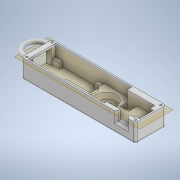
# Autodesk Inventor part: RespiraCheck-Enclosure-Top
Saved by Autodesk Inventor 2022 (Build 260153000, 153)
## iProperties
Created: 2022-04-28
Part Number: RespiraCheck-Enclosure-Top
Material: Generic
Document SubType Name: Modeling
Designer: incep
Density: 1 g/cm^3
Appearance: Default
Author: incep
Autodesk Inventor part; units mm, degrees
ref_plane "YZ Plane" through (0, 0, 0) normal (1, 0, 0) x (0, 1, 0)
ref_plane "XZ Plane" through (0, 0, 0) normal (0, 1, 0) x (-1, 0, 0)
ref_plane "XY Plane" through (0, 0, 0) normal (0, 0, 1) x (1, 0, 0)
sketch "Sketch1" plane through (0, 0, 0) normal (0, 1, 0) x (-1, 0, 0)
  line L0 (56, 15) -> (-56, 15)
  line L1 (-56, 15) -> (-56, -15)
  line L2 (-56, -15) -> (56, -15)
  line L3 (56, -15) -> (56, 15)
  point P0 (0, 0)
  point P1 (-56, 0)
  point P2 (0, -15)
  dimension "d0" = 30
  dimension "d1" = 112
  constraints: 8 end point, 2 midpoint, 2 parallel, 1 horizontal, 1 horizontal alignment, 1 perpendicular, 1 vertical alignment
  measures "d0" distance of L2.end L0.start
  measures "d1" distance of L1.end L2.end
extrude "Extrusion1" add sketch "Sketch1" along normal blind 19
sketch "Sketch2" plane through (0, 19, 0) normal (0, 1, 0) x (1, 0, 0)
  circle A0 centre (-53.5, 12.5) radius 2.5 construction
  line L0 (56, 15) -> (-56, 15) construction
  line L1 (-56, 15) -> (-56, -15) construction
  circle A1 centre (-53.5, -12.5) radius 2.5 construction
  circle A2 centre (53.5, 12.5) radius 2.5 construction
  circle A3 centre (53.5, -12.5) radius 2.5 construction
  line L2 (-56, -15) -> (56, -15) construction
  line L3 (56, -15) -> (56, 15) construction
  line L4 (-51, 13.6) -> (-3, 13.6)
  line L5 (-3, -13.6) -> (-51, -13.6)
  line L6 (-51, -13.6) -> (-51, 13.6)
  line L7 (-3, 8) -> (0, 8)
  line L8 (0, 8) -> (0, -8)
  line L9 (0, -8) -> (-3, -8)
  line L10 (-3, -8) -> (-3, 8) construction
  line L11 (-3, 8) -> (0, 5)
  line L12 (-3, -8) -> (0, -5)
  line L13 (-3, 13.6) -> (-3, 8)
  line L14 (-3, -8) -> (-3, -13.6)
  circle A4 centre (-53.5, 12.5) radius 1
  circle A5 centre (-53.5, -12.5) radius 1
  circle A6 centre (53.5, 12.5) radius 1
  circle A7 centre (53.5, -12.5) radius 1
  point P0 (0, 0)
  point P1 (-2, 0)
  point P2 (0, 0)
  point P3 (-51, 0)
  dimension "d4" = 5
  dimension "d5" = 5
  dimension "d6" = 5
  dimension "d7" = 5
  dimension "d8" = 27.2
  dimension "d10" = 3
  dimension "d11" = 16
  dimension "d14" = 48
  dimension "d15" = 45
  dimension "d16" = 45
  dimension "d64" = 2
  dimension "d65" = 2
  dimension "d66" = 2
  dimension "d67" = 2
  constraints: 22 end point, 9 tangent, 8 centre point, 5 coincident, 5 parallel, 3 perpendicular, 2 collinear, 2 horizontal, 2 midpoint, 2 point on line, 1 horizontal alignment
  measures "d4" diameter of A0
  measures "d5" diameter of A1
  measures "d6" diameter of A2
  measures "d7" diameter of A3
  measures "d8" distance of L5.end L4.start
  measures "d10" distance of L7.start L7.end
  measures "d11" distance of L7.end L8.end
  measures "d14" distance between parallel lines of L6 L13
  measures "d15" angle of L7 L11
  measures "d16" angle of L9 L12
  measures "d64" diameter of A4
  measures "d65" diameter of A5
  measures "d66" diameter of A6
  measures "d67" diameter of A7
extrude "Extrusion2" cut sketch "Sketch2" against normal blind 11.5 contours L4 L13 L11 L8 L12 L14 L5 L6 | A4 | A5 | A6 | A7
sketch "Sketch3" plane through (0, 7.5, 0) normal (0, 1, 0) x (1, 0, 0)
  line L0 (-3, 10) -> (-3, -10)
  line L1 (-51, -10) -> (-51, 10)
  line L2 (-51, -13.6) -> (-51, 13.6) projected
  line L3 (-3, 13.6) -> (-3, 8) projected
  line L4 (-10, -10) -> (-10, -13.6)
  line L5 (-10, -13.6) -> (-44, -13.6)
  line L6 (-44, -13.6) -> (-44, -10)
  line L7 (-3, -8) -> (-3, -13.6) projected
  line L8 (-3, -10) -> (-10, -10)
  line L9 (-44, -10) -> (-51, -10)
  line L10 (-51, 10) -> (-44, 10)
  line L11 (-10, 10) -> (-3, 10)
  line L12 (-51, 13.6) -> (-3, 13.6) projected
  line L13 (-9, 10) -> (-9, 13.6)
  line L14 (-9, 13.6) -> (-44, 13.6)
  line L15 (-44, 13.6) -> (-44, 10)
  point P0 (0, 0)
  point P1 (-3, 0)
  point P2 (-44, 13.6)
  dimension "d20" = 7
  dimension "d21" = 7
  constraints: 24 end point, 7 parallel, 3 point on line, 2 collinear, 2 horizontal, 2 perpendicular, 1 horizontal alignment, 1 midpoint
  measures "d20" distance between parallel lines of L4 L7
  measures "d21" distance between parallel lines of L2 L6
extrude "Extrusion3" cut sketch "Sketch3" against normal blind 5.5 contours L0 L8 L4 L5 L6 L9 L1 L10 L15 L12 L13 L11
sketch "Sketch4" plane through (0, 2, 0) normal (0, 1, 0) x (1, 0, 0)
  line L0 (-32, 5.1) -> (-8, 5.1)
  line L1 (-8, 5.1) -> (-8, -8.9)
  line L2 (-8, -8.9) -> (-32, -8.9)
  line L3 (-32, -8.9) -> (-32, 5.1)
  line L4 (-3, 8) -> (-3, -8) projected
  line L5 (-51, 13.6) -> (-3, 13.6) projected
  line L6 (-3, -13.6) -> (-51, -13.6) projected
  point P0 (0, 0)
  dimension "d24" = 5
  dimension "d25" = 8.5
  dimension "d26" = 4.7
  dimension "d27" = 24
  constraints: 8 end point, 2 parallel, 1 horizontal, 1 perpendicular
  measures "d24" distance between parallel lines of L4 L1
  measures "d25" distance between parallel lines of L0 L5
  measures "d26" distance between parallel lines of L6 L2
  measures "d27" distance between parallel lines of L3 L1
extrude "Extrusion4" cut sketch "Sketch4" against normal blind 2
sketch "Sketch5" plane through (0, 19, 0) normal (0, 1, 0) x (1, 0, 0)
  line L0 (-51, 13.6) -> (-3, 13.6) projected
  line L1 (-3, 13.6) -> (24, 13.6)
  line L2 (24, 13.6) -> (24, -13.6)
  line L3 (24, -13.6) -> (-3, -13.6)
  line L4 (-3, -13.6) -> (-3, 13.6)
  circle A0 centre (53.5, 12.5) radius 2.5 construction
  circle A1 centre (53.5, -12.5) radius 2.5 construction
  line L5 (-3, -13.6) -> (-51, -13.6) projected
  line L6 (0, 5) -> (0, -5) projected
  point P0 (0, 0)
  dimension "d43" = 24
  constraints: 8 end point, 2 parallel, 1 collinear, 1 horizontal, 1 perpendicular
  measures "d43" distance between parallel lines of L2 L6
extrude "Extrusion5" cut sketch "Sketch5" against normal blind 10.5
sketch "Sketch6" plane through (0, 8.5, 0) normal (0, 1, 0) x (1, 0, 0)
  circle A0 centre (12, 0) radius 10.1
  line L0 (0, -5) -> (0, 5) projected
  point P0 (0, 0)
  dimension "d32" = 20.2
  dimension "d33" = 12
  constraints: 1 centre point, 1 horizontal alignment
  measures "d32" diameter of A0
  measures "d33" distance from line of L0 A0.centre
extrude "Extrusion6" cut sketch "Sketch6" against normal blind 6.5
sketch "Sketch7" plane through (12, 2, 0) normal (0, 1, 0) x (1, 0, 0)
  circle A0 centre (0, 0) radius 10.1 projected
  circle A1 centre (0, 0) radius 6.5
  point P0 (-12, 0)
  dimension "d36" = 13
  constraints: 1 centre point, 1 coincident
  measures "d36" diameter of A1
extrude "Extrusion7" cut sketch "Sketch7" against normal blind 2 contours A1
sketch "Sketch8" plane through (0, 19, 0) normal (0, 1, 0) x (1, 0, 0)
  line L0 (24, 9.15) -> (51.1, 9.15)
  line L1 (51.1, 9.15) -> (51.1, -11.15)
  line L2 (51.1, -11.15) -> (24, -11.15)
  line L3 (24, -11.15) -> (24, 9.15)
  circle A0 centre (12, 0) radius 10.1 projected
  line L4 (24, -1) -> (51.1, -1) construction
  line L5 (24, 13.6) -> (24, -13.6) projected
  line L6 (51.1, 4.35) -> (54.6, 4.35)
  line L7 (54.6, 4.35) -> (54.6, -9.65)
  line L8 (54.6, -9.65) -> (51.1, -9.65)
  line L9 (51.1, -9.65) -> (51.1, 4.35)
  point P0 (0, 0)
  dimension "d39" = 20.3
  dimension "d42" = 1
  dimension "d46" = 27.1
  dimension "d47" = 14
  dimension "d48" = 3.5
  dimension "d49" = 1.5
  constraints: 18 end point, 4 parallel, 2 collinear, 2 horizontal, 2 midpoint, 2 perpendicular
  measures "d39" distance of L2.end L0.start
  measures "d42" vertical distance of L4.start A0.centre
  measures "d46" distance between parallel lines of L1 L3
  measures "d47" distance of L6.end L7.end
  measures "d48" distance of L6.start L6.end
  measures "d49" distance from line of L1.end L8
extrude "Extrusion8" cut sketch "Sketch8" against normal blind 9 contours L0 L1 L2 L3 | L6 L7 L8 L1
sketch "Sketch9" plane through (0, 10, 0) normal (0, 1, 0) x (1, 0, 0)
  line L0 (24, 9.15) -> (34, 9.15)
  line L1 (34, 9.15) -> (34, 0.15)
  line L2 (34, 0.15) -> (24, 0.15)
  line L3 (24, 0.15) -> (24, 9.15)
  line L4 (24, 9.15) -> (51.1, 9.15) projected
  line L5 (24, -11.15) -> (24, 9.15) projected
  point P0 (0, 0)
  dimension "d50" = 10
  dimension "d51" = 9
  constraints: 8 end point, 2 collinear, 2 parallel, 1 horizontal, 1 perpendicular
  measures "d50" distance of L1.end L2.end
  measures "d51" distance of L0.end L1.end
extrude "Extrusion9" cut sketch "Sketch9" against normal blind 10.5
sketch "Sketch10" plane through (51.1, 19, 11.15) normal (0, 0, -1) x (-1, 0, 0)
  line L0 (4, 0) -> (14, 0)
  line L1 (14, 0) -> (14, -9)
  line L2 (14, -9) -> (4, -9)
  line L3 (4, -9) -> (4, 0)
  line L4 (0, 0) -> (0, -9) projected
  line L5 (0, 0) -> (27.1, 0) projected
  line L6 (0, -9) -> (27.1, -9) projected
  point P0 (51.1, -19)
  dimension "d54" = 4
  dimension "d55" = 10
  constraints: 8 end point, 2 collinear, 2 parallel, 1 horizontal, 1 perpendicular
  measures "d54" distance between parallel lines of L4 L3
  measures "d55" distance between parallel lines of L1 L3
extrude "Extrusion10" cut sketch "Sketch10" against normal through all contours L0 L1 L2 L3
sketch "Sketch11" plane through (-56, 0, -15) normal (-1, 0, 0) x (0, 0, 1)
  line L0 (6, 17) -> (24, 17)
  line L1 (24, 17) -> (24, 2)
  line L2 (24, 2) -> (6, 2)
  line L3 (6, 2) -> (6, 17)
  line L4 (30, 0) -> (30, 19) projected
  line L5 (0, 0) -> (0, 19) projected
  line L6 (0, 0) -> (30, 0) projected
  line L7 (0, 19) -> (30, 19) projected
  point P0 (15, 0)
  dimension "d58" = 6
  dimension "d59" = 6
  dimension "d60" = 2
  dimension "d61" = 2
  constraints: 8 end point, 2 parallel, 1 horizontal, 1 perpendicular
  measures "d58" distance between parallel lines of L4 L1
  measures "d59" distance between parallel lines of L5 L3
  measures "d60" distance between parallel lines of L6 L2
  measures "d61" distance between parallel lines of L7 L0
extrude "Extrusion11" cut sketch "Sketch11" against normal up to surface (5 mm away) contours L0 L1 L2 L3
sketch "Sketch12" plane through (0, 0, 0) normal (0, -1, 0) x (1, 0, 0)
  line L0 (-45.861, -11.1947) -> (-45.861, 30.7358) construction
  line L1 (-45.861, 30.7358) -> (-41.9267, 30.7358) construction
  line L2 (-41.9267, 30.7358) -> (-41.9267, -11.1947) construction
  line L3 (-41.9267, -11.1947) -> (-45.861, -11.1947) construction
  line L4 (-43.2644, -9.2745) -> (-44.1875, -9.9511)
  spline S0 degree 2 poles (-44.1875, -9.9511) (-44.274, -9.6153) (-44.6708, -9.2974) (-44.9632, -9.2974) knots 0 0 0 1 2 2 2
  spline S1 degree 2 poles (-44.9632, -9.2974) (-45.154, -9.2974) (-45.4693, -9.4322) (-45.5787, -9.5619) knots 0 0 0 1 2 2 2
  spline S2 degree 2 poles (-45.5787, -9.5619) (-45.6804, -9.6789) (-45.7644, -9.9943) (-45.7644, -10.2435) knots 0 0 0 1 2 2 2
  line L5 (-45.7644, -10.2435) -> (-45.7644, -10.9633)
  line L6 (-45.7644, -10.9633) -> (-43.2644, -10.9633)
  line L7 (-43.2644, -10.9633) -> (-43.2644, -10.5004)
  line L8 (-43.2644, -10.5004) -> (-44.2232, -10.5004)
  line L9 (-44.2232, -10.5004) -> (-43.2644, -9.8468)
  line L10 (-43.2644, -9.8468) -> (-43.2644, -9.2745)
  spline S3 degree 2 poles (-44.9505, -9.7654) (-44.7521, -9.7629) (-44.569, -10.007) (-44.5716, -10.274) knots 0 0 0 1 2 2 2
  line L11 (-44.5716, -10.274) -> (-44.5716, -10.5004)
  line L12 (-44.5716, -10.5004) -> (-45.3218, -10.5004)
  line L13 (-45.3218, -10.5004) -> (-45.3218, -10.2944)
  spline S4 degree 2 poles (-45.3218, -10.2944) (-45.3218, -10.0782) (-45.2277, -9.8468) (-45.0624, -9.7629) (-44.9505, -9.7654) knots 0 0 0 1 2 3 3 3
  spline S5 degree 2 poles (-44.1748, -7.1764) (-44.4673, -7.1789) (-44.92, -7.4282) (-45.1794, -7.8631) (-45.182, -8.1454) knots 0 0 0 1 2 3 3 3
  spline S6 degree 2 poles (-45.182, -8.1454) (-45.1794, -8.4226) (-44.9175, -8.8676) (-44.4749, -9.1296) (-44.1952, -9.1321) knots 0 0 0 1 2 3 3 3
  spline S7 degree 2 poles (-44.1952, -9.1321) (-43.918, -9.1296) (-43.4805, -8.8625) (-43.2237, -8.4073) (-43.2211, -8.1174) knots 0 0 0 1 2 3 3 3
  spline S8 degree 2 poles (-43.2211, -8.1174) (-43.2211, -7.9266) (-43.3585, -7.5655) (-43.6255, -7.2908) (-43.8188, -7.2247) knots 0 0 0 1 2 3 3 3
  line L14 (-43.8188, -7.2247) -> (-43.8188, -7.7155)
  spline S9 degree 2 poles (-43.8188, -7.7155) (-43.7196, -7.7995) (-43.6331, -7.9902) (-43.6331, -8.1276) knots 0 0 0 1 2 2 2
  spline S10 degree 2 poles (-43.6331, -8.1276) (-43.6357, -8.331) (-43.8315, -8.6031) (-44.0019, -8.6464) knots 0 0 0 1 2 2 2
  line L15 (-44.0019, -8.6464) -> (-44.0019, -7.1942)
  spline S11 degree 2 poles (-44.0019, -7.1942) (-44.0477, -7.184) (-44.1265, -7.1764) (-44.1748, -7.1764) knots 0 0 0 1 2 2 2
  line L16 (-44.3986, -7.6214) -> (-44.3986, -8.6591)
  spline S12 degree 2 poles (-44.3986, -8.6591) (-44.5792, -8.6057) (-44.77, -8.3386) (-44.77, -8.1377) knots 0 0 0 1 2 2 2
  spline S13 degree 2 poles (-44.77, -8.1377) (-44.77, -7.9292) (-44.5792, -7.6647) (-44.3986, -7.6214) knots 0 0 0 1 2 2 2
  spline S14 degree 2 poles (-43.8595, -5.6479) (-44.0655, -5.6428) (-44.3198, -5.8793) (-44.4088, -6.1693) knots 0 0 0 1 2 2 2
  spline S15 degree 2 poles (-44.4088, -6.1693) (-44.4546, -6.3193) (-44.5105, -6.4566) (-44.5639, -6.4897) (-44.6123, -6.4872) knots 0 0 0 1 2 3 3 3
  spline S16 degree 2 poles (-44.6123, -6.4872) (-44.6809, -6.4846) (-44.77, -6.3905) (-44.77, -6.3142) knots 0 0 0 1 2 2 2
  spline S17 degree 2 poles (-44.77, -6.3142) (-44.77, -6.243) (-44.6937, -6.154) (-44.6224, -6.1387) knots 0 0 0 1 2 2 2
  line L17 (-44.6224, -6.1387) -> (-44.6224, -5.6988)
  spline S18 degree 2 poles (-44.6224, -5.6988) (-44.7979, -5.7089) (-45.0472, -5.8819) (-45.182, -6.154) (-45.182, -6.3142) knots 0 0 0 1 2 3 3 3
  spline S19 degree 2 poles (-45.182, -6.3142) (-45.1769, -6.5813) (-44.8564, -6.9297) (-44.6123, -6.9373) knots 0 0 0 1 2 2 2
  spline S20 degree 2 poles (-44.6123, -6.9373) (-44.4088, -6.9399) (-44.1469, -6.6932) (-44.0553, -6.416) knots 0 0 0 1 2 2 2
  spline S21 degree 2 poles (-44.0553, -6.416) (-44.007, -6.2684) (-43.9383, -6.1311) (-43.8696, -6.0955) (-43.8162, -6.098) knots 0 0 0 1 2 3 3 3
  spline S22 degree 2 poles (-43.8162, -6.098) (-43.7349, -6.1006) (-43.6357, -6.2125) (-43.6331, -6.3015) knots 0 0 0 1 2 2 2
  spline S23 degree 2 poles (-43.6331, -6.3015) (-43.6331, -6.3982) (-43.7399, -6.5202) (-43.8595, -6.5507) knots 0 0 0 1 2 2 2
  line L18 (-43.8595, -6.5507) -> (-43.8595, -7.006)
  spline S24 degree 2 poles (-43.8595, -7.006) (-43.5339, -6.9653) (-43.2211, -6.6016) (-43.2211, -6.3168) knots 0 0 0 1 2 2 2
  spline S25 degree 2 poles (-43.2211, -6.3168) (-43.2237, -6.1286) (-43.3915, -5.8259) (-43.6789, -5.6504) (-43.8595, -5.6479) knots 0 0 0 1 2 3 3 3
  spline S26 degree 2 poles (-44.2079, -3.4378) (-44.4927, -3.4404) (-44.9302, -3.6794) (-45.1794, -4.0991) (-45.182, -4.3712) knots 0 0 0 1 2 3 3 3
  spline S27 degree 2 poles (-45.182, -4.3712) (-45.182, -4.5619) (-45.0446, -4.8773) (-44.9175, -4.9867) knots 0 0 0 1 2 2 2
  line L19 (-44.9175, -4.9867) -> (-45.1387, -4.9867)
  line L20 (-45.1387, -4.9867) -> (-45.1387, -5.3987)
  line L21 (-45.1387, -5.3987) -> (-42.6387, -5.3987)
  line L22 (-42.6387, -5.3987) -> (-42.6387, -4.9485)
  line L23 (-42.6387, -4.9485) -> (-43.4398, -4.9485)
  spline S28 degree 2 poles (-43.4398, -4.9485) (-43.3279, -4.8239) (-43.2211, -4.5441) (-43.2211, -4.3737) knots 0 0 0 1 2 2 2
  spline S29 degree 2 poles (-43.2211, -4.3737) (-43.2237, -4.1016) (-43.478, -3.6794) (-43.9205, -3.4404) (-44.2079, -3.4378) knots 0 0 0 1 2 3 3 3
  spline S30 degree 2 poles (-44.1977, -3.8905) (-43.9536, -3.8956) (-43.6382, -4.1932) (-43.6331, -4.4221) knots 0 0 0 1 2 2 2
  spline S31 degree 2 poles (-43.6331, -4.4221) (-43.6382, -4.6637) (-43.9536, -4.9714) (-44.2054, -4.9765) knots 0 0 0 1 2 2 2
  spline S32 degree 2 poles (-44.2054, -4.9765) (-44.452, -4.9714) (-44.7649, -4.6662) (-44.77, -4.4271) knots 0 0 0 1 2 2 2
  spline S33 degree 2 poles (-44.77, -4.4271) (-44.7649, -4.1957) (-44.447, -3.8956) (-44.1977, -3.8905) knots 0 0 0 1 2 2 2
  line L24 (-43.2644, -2.7155) -> (-45.1387, -2.7155)
  line L25 (-45.1387, -2.7155) -> (-45.1387, -3.1657)
  line L26 (-45.1387, -3.1657) -> (-43.2644, -3.1657)
  line L27 (-43.2644, -3.1657) -> (-43.2644, -2.7155)
  line L28 (-45.4083, -2.713) -> (-45.8585, -2.713)
  line L29 (-45.8585, -2.713) -> (-45.8585, -3.1632)
  line L30 (-45.8585, -3.1632) -> (-45.4083, -3.1632)
  line L31 (-45.4083, -3.1632) -> (-45.4083, -2.713)
  line L32 (-44.7496, -1.5024) -> (-45.182, -1.5024)
  line L33 (-45.182, -1.5024) -> (-45.182, -1.5355)
  spline S34 degree 2 poles (-45.182, -1.5355) (-45.1845, -1.6754) (-45.0828, -1.8559) (-44.9556, -1.9424) knots 0 0 0 1 2 2 2
  line L34 (-44.9556, -1.9424) -> (-45.1387, -1.9424)
  line L35 (-45.1387, -1.9424) -> (-45.1387, -2.3544)
  line L36 (-45.1387, -2.3544) -> (-43.2644, -2.3544)
  line L37 (-43.2644, -2.3544) -> (-43.2644, -1.9043)
  line L38 (-43.2644, -1.9043) -> (-44.3071, -1.9043)
  spline S35 degree 2 poles (-44.3071, -1.9043) (-44.5233, -1.9043) (-44.7445, -1.7059) (-44.7496, -1.5024) knots 0 0 0 1 2 2 2
  line L39 (-43.2644, 0.6263) -> (-45.1387, 0.6263)
  line L40 (-45.1387, 0.6263) -> (-45.1387, 0.2117)
  line L41 (-45.1387, 0.2117) -> (-44.8869, 0.2117)
  spline S36 degree 2 poles (-44.8869, 0.2117) (-45.0421, 0.0973) (-45.182, -0.1977) (-45.182, -0.3987) knots 0 0 0 1 2 2 2
  spline S37 degree 2 poles (-45.182, -0.3987) (-45.1794, -0.6784) (-44.9276, -1.1057) (-44.4826, -1.3498) (-44.1952, -1.3524) knots 0 0 0 1 2 3 3 3
  spline S38 degree 2 poles (-44.1952, -1.3524) (-43.9103, -1.3498) (-43.4729, -1.1082) (-43.2237, -0.686) (-43.2211, -0.4088) knots 0 0 0 1 2 3 3 3
  spline S39 degree 2 poles (-43.2211, -0.4088) (-43.2211, -0.213) (-43.3585, 0.082) (-43.5085, 0.2117) knots 0 0 0 1 2 2 2
  line L42 (-43.5085, 0.2117) -> (-43.2644, 0.2117)
  line L43 (-43.2644, 0.2117) -> (-43.2644, 0.6263)
  spline S40 degree 2 poles (-44.1875, 0.199) (-43.9485, 0.1965) (-43.6382, -0.0858) (-43.6331, -0.3453) knots 0 0 0 1 2 2 2
  spline S41 degree 2 poles (-43.6331, -0.3453) (-43.6357, -0.5945) (-43.9358, -0.8971) (-44.185, -0.8997) knots 0 0 0 1 2 2 2
  spline S42 degree 2 poles (-44.185, -0.8997) (-44.4444, -0.8946) (-44.7649, -0.597) (-44.77, -0.3529) knots 0 0 0 1 2 2 2
  spline S43 degree 2 poles (-44.77, -0.3529) (-44.7649, -0.1062) (-44.4495, 0.1939) (-44.1875, 0.199) knots 0 0 0 1 2 2 2
  line L44 (-43.9612, 3.3501) -> (-43.9612, 2.8058)
  spline S44 degree 2 poles (-43.9612, 2.8058) (-43.8035, 2.6558) (-43.6662, 2.3633) (-43.6687, 2.1878) knots 0 0 0 1 2 2 2
  spline S45 degree 2 poles (-43.6687, 2.1878) (-43.6713, 1.9538) (-43.9002, 1.5749) (-44.2842, 1.3511) (-44.5182, 1.3485) knots 0 0 0 1 2 3 3 3
  spline S46 degree 2 poles (-44.5182, 1.3485) (-44.7572, 1.3511) (-45.1362, 1.5647) (-45.3574, 1.936) (-45.36, 2.1776) knots 0 0 0 1 2 3 3 3
  spline S47 degree 2 poles (-45.36, 2.1776) (-45.3625, 2.3938) (-45.2099, 2.7092) (-45.0472, 2.8338) knots 0 0 0 1 2 2 2
  line L45 (-45.0472, 2.8338) -> (-45.0472, 3.3501)
  spline S48 degree 2 poles (-45.0472, 3.3501) (-45.4108, 3.1797) (-45.805, 2.5566) (-45.8076, 2.1675) knots 0 0 0 1 2 2 2
  spline S49 degree 2 poles (-45.8076, 2.1675) (-45.8025, 1.8089) (-45.4592, 1.229) (-44.8793, 0.8857) (-44.5233, 0.8806) knots 0 0 0 1 2 3 3 3
  spline S50 degree 2 poles (-44.5233, 0.8806) (-44.1596, 0.8857) (-43.5721, 1.2341) (-43.2262, 1.8267) (-43.2211, 2.198) knots 0 0 0 1 2 3 3 3
  spline S51 degree 2 poles (-43.2211, 2.198) (-43.2262, 2.5871) (-43.6153, 3.1975) (-43.9612, 3.3501) knots 0 0 0 1 2 2 2
  line L46 (-43.2644, 5.26) -> (-44.3249, 5.26)
  spline S52 degree 2 poles (-44.3249, 5.26) (-44.7827, 5.255) (-45.1896, 4.8658) (-45.187, 4.525) knots 0 0 0 1 2 2 2
  spline S53 degree 2 poles (-45.187, 4.525) (-45.187, 4.3826) (-45.1006, 4.1486) (-45.0116, 4.0495) knots 0 0 0 1 2 2 2
  line L47 (-45.0116, 4.0495) -> (-45.7644, 4.0495)
  line L48 (-45.7644, 4.0495) -> (-45.7644, 3.5993)
  line L49 (-45.7644, 3.5993) -> (-43.2644, 3.5993)
  line L50 (-43.2644, 3.5993) -> (-43.2644, 4.0495)
  line L51 (-43.2644, 4.0495) -> (-44.2155, 4.0495)
  spline S54 degree 2 poles (-44.2155, 4.0495) (-44.5207, 4.0495) (-44.775, 4.2504) (-44.77, 4.4437) knots 0 0 0 1 2 2 2
  spline S55 degree 2 poles (-44.77, 4.4437) (-44.7725, 4.642) (-44.5131, 4.8124) (-44.2232, 4.8099) knots 0 0 0 1 2 2 2
  line L52 (-44.2232, 4.8099) -> (-43.2644, 4.8099)
  line L53 (-43.2644, 4.8099) -> (-43.2644, 5.26)
  spline S56 degree 2 poles (-44.1748, 7.5032) (-44.4673, 7.5006) (-44.92, 7.2514) (-45.1794, 6.8165) (-45.182, 6.5342) knots 0 0 0 1 2 3 3 3
  spline S57 degree 2 poles (-45.182, 6.5342) (-45.1794, 6.257) (-44.9175, 5.8119) (-44.4749, 5.55) (-44.1952, 5.5474) knots 0 0 0 1 2 3 3 3
  spline S58 degree 2 poles (-44.1952, 5.5474) (-43.918, 5.55) (-43.4805, 5.817) (-43.2237, 6.2722) (-43.2211, 6.5622) knots 0 0 0 1 2 3 3 3
  spline S59 degree 2 poles (-43.2211, 6.5622) (-43.2211, 6.7529) (-43.3585, 7.1141) (-43.6255, 7.3887) (-43.8188, 7.4549) knots 0 0 0 1 2 3 3 3
  line L54 (-43.8188, 7.4549) -> (-43.8188, 6.964)
  spline S60 degree 2 poles (-43.8188, 6.964) (-43.7196, 6.8801) (-43.6331, 6.6893) (-43.6331, 6.552) knots 0 0 0 1 2 2 2
  spline S61 degree 2 poles (-43.6331, 6.552) (-43.6357, 6.3485) (-43.8315, 6.0764) (-44.0019, 6.0332) knots 0 0 0 1 2 2 2
  line L55 (-44.0019, 6.0332) -> (-44.0019, 7.4854)
  spline S62 degree 2 poles (-44.0019, 7.4854) (-44.0477, 7.4955) (-44.1265, 7.5032) (-44.1748, 7.5032) knots 0 0 0 1 2 2 2
  line L56 (-44.3986, 7.0581) -> (-44.3986, 6.0205)
  spline S63 degree 2 poles (-44.3986, 6.0205) (-44.5792, 6.0739) (-44.77, 6.3409) (-44.77, 6.5418) knots 0 0 0 1 2 2 2
  spline S64 degree 2 poles (-44.77, 6.5418) (-44.77, 6.7504) (-44.5792, 7.0149) (-44.3986, 7.0581) knots 0 0 0 1 2 2 2
  line L57 (-43.8798, 9.642) -> (-43.8798, 9.1359)
  spline S65 degree 2 poles (-43.8798, 9.1359) (-43.7501, 9.052) (-43.6331, 8.846) (-43.6331, 8.7087) knots 0 0 0 1 2 2 2
  spline S66 degree 2 poles (-43.6331, 8.7087) (-43.6382, 8.4696) (-43.9536, 8.1695) (-44.2054, 8.1644) knots 0 0 0 1 2 2 2
  spline S67 degree 2 poles (-44.2054, 8.1644) (-44.4546, 8.1695) (-44.7649, 8.462) (-44.77, 8.6985) knots 0 0 0 1 2 2 2
  spline S68 degree 2 poles (-44.77, 8.6985) (-44.77, 8.8511) (-44.6428, 9.0673) (-44.5131, 9.1359) knots 0 0 0 1 2 2 2
  line L58 (-44.5131, 9.1359) -> (-44.5131, 9.642)
  spline S69 degree 2 poles (-44.5131, 9.642) (-44.8361, 9.5276) (-45.1794, 9.024) (-45.182, 8.6985) knots 0 0 0 1 2 2 2
  spline S70 degree 2 poles (-45.182, 8.6985) (-45.1794, 8.4187) (-44.9225, 7.9737) (-44.48, 7.7143) (-44.2003, 7.7117) knots 0 0 0 1 2 3 3 3
  spline S71 degree 2 poles (-44.2003, 7.7117) (-43.9256, 7.7143) (-43.4856, 7.9813) (-43.2237, 8.4315) (-43.2211, 8.7112) knots 0 0 0 1 2 3 3 3
  spline S72 degree 2 poles (-43.2211, 8.7112) (-43.2237, 9.0418) (-43.5645, 9.5225) (-43.8798, 9.642) knots 0 0 0 1 2 2 2
  line L59 (-43.2644, 11.6512) -> (-44.2206, 10.873)
  line L60 (-44.2206, 10.873) -> (-45.1387, 11.5444)
  line L61 (-45.1387, 11.5444) -> (-45.1387, 11.0052)
  line L62 (-45.1387, 11.0052) -> (-44.2562, 10.4075)
  line L63 (-44.2562, 10.4075) -> (-45.7644, 10.4075)
  line L64 (-45.7644, 10.4075) -> (-45.7644, 9.9574)
  line L65 (-45.7644, 9.9574) -> (-43.2644, 9.9574)
  line L66 (-43.2644, 9.9574) -> (-43.2644, 10.4075)
  line L67 (-43.2644, 10.4075) -> (-44.1418, 10.4075)
  line L68 (-44.1418, 10.4075) -> (-43.2644, 11.0459)
  line L69 (-43.2644, 11.0459) -> (-43.2644, 11.6512)
  point P0 (0, 0)
  constraints: 2 other
extrude "Extrusion12" cut sketch "Sketch12" against normal blind 1
chamfer "Chamfer1" distance 2 angle 45 9 edges at (-20, 0, 8.9) (-8, 0, 1.9) (-20, 0, -5.1) (-32, 0, 1.9) (5.5, 0, 0) (29, 0, -0.15) (24, 0, -4.65) (34, 0, -4.65) (29, 0, -9.15)
chamfer "Chamfer2" distance 2 angle 45 3 edges at (37.1, 14.5, 15) (42.1, 10, 15) (47.1, 14.5, 15)
fillet "Fillet1" radius 2 17 edges at (-20, 0, 10.8999) (-6.0001, 0, 1.9) (-20, 0, -7.0999) (-33.9999, 0, 1.9) (3.5001, 0, 0) (29, 0, 1.8499) (22.0001, 0, -4.65) (29, 0, -11.1499) (35.9999, 0, -4.65) (0, 0, -15) (56, 9.5, -15) (56, 0, 0) (0, 0, 15) (-56, 0, 0) (-56, 9.5, -15) (-56, 9.5, 15) (56, 9.5, 15)
sketch "Sketch13" plane through (-56, 17, -10) normal (-1, 0, 0) x (0, 0, 1)
  circle A0 centre (21, 0) radius 2
  line L0 (23, 2) -> (23, -15) projected
  line L1 (-3, 2) -> (23, 2) projected
  circle A1 centre (-1, 0) radius 2
  line L2 (-3, -15) -> (-3, 2) projected
  point P0 (10, -17)
  dimension "d77" = 4
  dimension "d78" = 2
  dimension "d79" = 4
  dimension "d80" = 2
  constraints: 2 centre point, 2 tangent
  measures "d77" diameter of A0
  measures "d78" distance from line of L0 A0.centre
  measures "d79" diameter of A1
  measures "d80" distance from line of L2 A1.centre
ref_plane "Work Plane1" through (-56, 17, 11) normal (0, 1, 0) x (1, 0, 0)
sketch "Sketch14" plane through (-56, 17, 11) normal (0, 1, 0) x (1, 0, 0)
  line L0 (0, 2) -> (0, -2) projected
  line L1 (0, 20) -> (0, 2) projected
  arc A0 (0, 22) -> (0, 0) centre (0, 11) ccw
  line L2 (0, 24) -> (0, 20) construction
  line L3 (0, 0) -> (0, 22) construction
  point P0 (56, 11)
  constraints: 3 midpoint, 2 end point, 2 point on circle, 1 centre point
sweep "Sweep1" add profiles "Sketch13" path "Sketch14" path curves A0 contours A0
body "Solid1"
